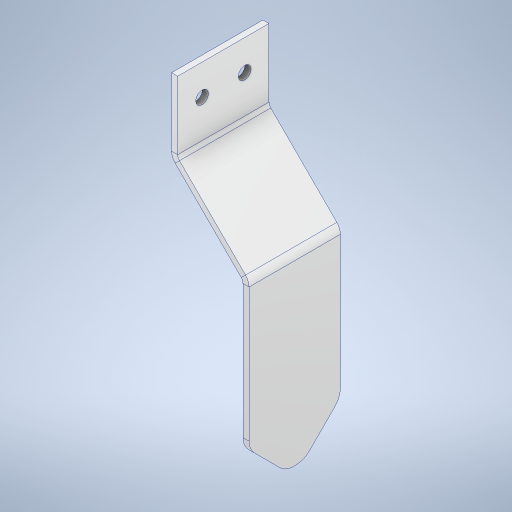
# Autodesk Inventor part: RSFF_tip_metal_1
Saved by Autodesk Inventor 2023 (Build 270158000, 158)
## iProperties
Created: 2023-06-24
Part Number: RSFF_tip_metal_1
Material: アルミニウム 6061
Document SubType Name: Sheet Metal
Designer: user
Density: 2.7 g/cm^3
Sheet Metal Rule: Default_mm
Appearance: アルミニウム - フラット
Author: user
Autodesk Inventor part; units mm, degrees
ref_plane "YZ Plane" through (0, 0, 0) normal (1, 0, 0) x (0, 1, 0)
ref_plane "XZ Plane" through (0, 0, 0) normal (0, 1, 0) x (-1, 0, 0)
ref_plane "XY Plane" through (0, 0, 0) normal (0, 0, 1) x (1, 0, 0)
sketch "スケッチ1" plane through (0, 0, 0) normal (1, 0, 0) x (0, 1, 0)
  line L0 (0, 0) -> (-12, 0)
  line L1 (-12, 0) -> (-12, -15)
  line L2 (-12, -15) -> (0, -15)
  line L3 (0, -15) -> (0, 0)
  dimension "d0" = 12
  dimension "d1" = 15
  measures "d0" distance of L1.end L2.end
  measures "d1" distance of L0.end L1.end
extrude "プレート1" add sketch "スケッチ1" along normal blind 1
sketch "スケッチ2" plane through (0.7071, -11.2929, -15) normal (-0.7071068, -0.7071068, 0) x (0.7071068, -0.7071068, 0)
  line L0 (0, 15) -> (0, 0)
  line L1 (0, 0) -> (17, 0)
  line L2 (17, 0) -> (17, 15)
  line L3 (17, 15) -> (0, 15)
  constraints: 6 end point, 1 horizontal, 1 perpendicular, 1 vertical
edge flange "フランジ1" height 17 angle 45 thickness 1 bend radius 1 thickness toward (-0.7071068, -0.7071068, 0) relief tear relief width 1 relief depth 0.5 edges at (1, -12, -7.5) wall of the first edge with corners at (0.7071, -11.2929, 0) (0.7071, -11.2929, -15) (12.7279, -23.3137, -15) (12.7279, -23.3137, 0)
bend "曲げ1"
corner "コーナー1"
sketch "スケッチ3" plane through (11.7279, -23.3137, 0) normal (1, 0, 0) x (0, 1, 0)
  line L0 (0, -15) -> (0, 0)
  line L1 (0, 0) -> (-30, 0)
  line L2 (-30, 0) -> (-30, -15)
  line L3 (-30, -15) -> (0, -15)
  constraints: 6 end point, 1 horizontal, 1 perpendicular, 1 vertical
edge flange "フランジ2" height 30 angle 45 thickness 1 bend radius 1 thickness toward (1, 0, 0) relief tear relief width 1 relief depth 0.5 edges at (12.0208, -24.0208, -7.5) wall of the first edge with corners at (11.7279, -23.3137, -15) (11.7279, -23.3137, 0) (11.7279, -53.3137, 0) (11.7279, -53.3137, -15)
bend "曲げ2"
corner "コーナー2"
sketch "スケッチ4" plane through (12.7279, -53.3137, 0) normal (1, 0, 0) x (0, 0, -1)
  line L0 (15, 0) -> (0, 0) projected
  line L1 (0, 29.1716) -> (15, 29.1716) projected
  line L2 (0, 0) -> (15, 0)
  line L3 (15, 0) -> (15, 29.1716)
  line L4 (15, 29.1716) -> (0, 29.1716)
  line L5 (0, 29.1716) -> (0, 0)
  line L6 (0, 29.1716) -> (0, 0) projected
  line L7 (0, 6) -> (6, 0)
  line L8 (9, 0) -> (15, 6)
  line L9 (15, 29.1716) -> (15, 0) projected
  point P0 (0, 53.3137)
  dimension "d23" = 45
  dimension "d24" = 45
  dimension "d25" = 6
  dimension "d26" = 6
  constraints: 12 end point, 4 point on line, 2 parallel, 1 horizontal, 1 perpendicular
  measures "d23" angle of L7 L0
  measures "d24" angle of L0 L8
  measures "d25" distance from line of L3 L8.start
  measures "d26" distance from line of L7.end L5
extrude "切り取り1" cut sketch "スケッチ4" against normal blind 1 contours L0 L8 L3 | L0 L5 L7
fillet "コーナーR2" radius 3 4 edges at (12.2279, -47.3137, 0) (12.2279, -53.3137, -6) (12.2279, -53.3137, -9) (12.2279, -47.3137, -15)
sketch "スケッチ6" plane through (1, 0, 0) normal (1, 0, 0) x (0, 0, -1)
  line L0 (0, 0) -> (15, 0) projected
  line L1 (0, -11.1716) -> (0, 0) projected
  line L2 (15, 0) -> (15, -11.1716) projected
  point P0 (4, -5)
  point P1 (11, -5)
  point P2 (0, -5.5858)
  dimension "d40" = 5
  dimension "d41" = 5
  dimension "d42" = 4
  dimension "d43" = 4
  constraints: 1 midpoint
  measures "d40" distance from line of L0 point (4, -5)
  measures "d41" distance from line of L0 point (11, -5)
  measures "d42" horizontal distance of point (0, -5.586) point (4, -5)
  measures "d43" distance from line of L2 point (11, -5)
hole "穴2" at (1, -5, -4) at (1, -5, -11) direction (-1, 0, 0) diameter 2.1 end through all
equation "\"d26\" = d25"
equation "\"d27\" = Thickness"
equation "\"d49\" = Thickness"
equation "\"d2\" = Thickness"
equation "\"d3\" = BendReliefWidth"
equation "\"d4\" = BendReliefDepth"
equation "\"d5\" = MinimumRemnant"
equation "\"d6\" = TransitionRadius"
equation "\"d9\" = BendRadius"
equation "\"d10\" = CornerReliefSize"
equation "\"d11\" = GapSize"
equation "\"d12\" = JacobiRadiusSize"
equation "\"d13\" = BendReliefWidth"
equation "\"d14\" = BendReliefDepth"
equation "\"d15\" = MinimumRemnant"
equation "\"d16\" = TransitionRadius"
equation "\"d19\" = BendRadius"
equation "\"d20\" = CornerReliefSize"
equation "\"d21\" = GapSize"
equation "\"d22\" = JacobiRadiusSize"
equation "\"BendRadius\" = Thickness"
equation "\"BendReliefWidth\" = Thickness"
equation "\"BendReliefDepth\" = 0.5 * Thickness"
equation "\"CornerReliefSize\" = 4 * Thickness"
equation "\"MinimumRemnant\" = 2 * Thickness"
equation "\"TransitionRadius\" = BendRadius"
equation "\"JacobiRadiusSize\" = BendRadius"
equation "\"GapSize\" = Thickness"
equation "\"Thickness\" = 1"
